Autodesk Fusion 360 part; units mm, degrees
note: some values were not read from the file. Chosen so that the rebuilt part matches the saved one: a direction. Set by a fixed rule: which sketch regions a step uses.
(part 6 of 6)
  spline S38 degree 5 poles (-15.5097, -25.0741) (-15.5106, -25.0685) (-15.5125, -25.0573) (-15.5158, -25.0407) (-15.521, -25.0187) (-15.5286, -24.9914) (-15.537, -24.9643) (-15.5458, -24.9373) (-15.5549, -24.9103) (-15.5642, -24.8833) (-15.5737, -24.8564) (-15.5835, -24.8296) (-15.5935, -24.8028) (-15.604, -24.776) (-15.6148, -24.7494) (-15.6259, -24.7229) (-15.6374, -24.6964) (-15.6491, -24.67) (-15.661, -24.6436) (-15.6731, -24.6173) (-15.6855, -24.591) (-15.698, -24.5648) (-15.7108, -24.5387) (-15.7238, -24.5126) (-15.7371, -24.4866) (-15.7506, -24.4606) (-15.7643, -24.4347) (-15.7782, -24.4088) (-15.7922, -24.383) (-15.8065, -24.3573) (-15.821, -24.3316) (-15.8356, -24.3059) (-15.8505, -24.2803) (-15.8655, -24.2548) (-15.8807, -24.2293) (-15.8961, -24.2039) (-15.9116, -24.1785) (-15.9274, -24.1532) (-15.9433, -24.128) (-15.9594, -24.1028) (-15.9756, -24.0776) (-15.9921, -24.0525) (-16.0086, -24.0275) (-16.0254, -24.0025) (-16.0423, -23.9776) (-16.0594, -23.9527) (-16.0766, -23.9279) (-16.094, -23.9031) (-16.1115, -23.8784) (-16.1292, -23.8537) (-16.1471, -23.8291) (-16.1651, -23.8045) (-16.1832, -23.78) (-16.2015, -23.7556) (-16.22, -23.7312) (-16.2386, -23.7069) (-16.2573, -23.6826) (-16.2762, -23.6584) (-16.2952, -23.6342) (-16.3144, -23.6101) (-16.3337, -23.5861) (-16.3532, -23.5621) (-16.3728, -23.5381) (-16.3925, -23.5143) (-16.4124, -23.4904) (-16.4324, -23.4667) (-16.4525, -23.4429) (-16.4728, -23.4193) (-16.4932, -23.3957) (-16.5137, -23.3722) (-16.5344, -23.3487) (-16.5511, -23.3299) (-16.5636, -23.3159) (-16.572, -23.3066) (-16.5762, -23.3019) knots 0 0 0 0 0 0 0.01428571 0.02857143 0.04285714 0.05714286 0.07142857 0.08571429 0.1 0.11428571 0.12857143 0.14285714 0.15714286 0.17142857 0.18571429 0.2 0.21428571 0.22857143 0.24285714 0.25714286 0.27142857 0.28571429 0.3 0.31428571 0.32857143 0.34285714 0.35714286 0.37142857 0.38571429 0.4 0.41428571 0.42857143 0.44285714 0.45714286 0.47142857 0.48571429 0.5 0.51428571 0.52857143 0.54285714 0.55714286 0.57142857 0.58571429 0.6 0.61428571 0.62857143 0.64285714 0.65714286 0.67142857 0.68571429 0.7 0.71428571 0.72857143 0.74285714 0.75714286 0.77142857 0.78571429 0.8 0.81428571 0.82857143 0.84285714 0.85714286 0.87142857 0.88571429 0.9 0.91428571 0.92857143 0.94285714 0.95714286 0.97142857 0.98571429 1 1 1 1 1 1
  arc A78 (-16.5762, -23.3019) -> (-17.3581, -23.4928) centre (-13.5, -37.5997) ccw
  spline S39 degree 5 poles (-17.3581, -23.4928) (-17.3597, -23.4989) (-17.3628, -23.511) (-17.3675, -23.5292) (-17.3736, -23.5535) (-17.3812, -23.5839) (-17.3885, -23.6143) (-17.3958, -23.6446) (-17.4029, -23.675) (-17.4098, -23.7053) (-17.4166, -23.7356) (-17.4233, -23.7659) (-17.4298, -23.7962) (-17.4361, -23.8265) (-17.4424, -23.8567) (-17.4484, -23.887) (-17.4543, -23.9172) (-17.4601, -23.9474) (-17.4657, -23.9776) (-17.4711, -24.0078) (-17.4764, -24.0379) (-17.4815, -24.0681) (-17.4865, -24.0982) (-17.4914, -24.1283) (-17.496, -24.1584) (-17.5005, -24.1885) (-17.5049, -24.2185) (-17.509, -24.2485) (-17.5131, -24.2785) (-17.5169, -24.3085) (-17.5206, -24.3384) (-17.5241, -24.3684) (-17.5275, -24.3983) (-17.5306, -24.4281) (-17.5337, -24.458) (-17.5365, -24.4878) (-17.5391, -24.5176) (-17.5416, -24.5473) (-17.5439, -24.577) (-17.5461, -24.6067) (-17.548, -24.6364) (-17.5498, -24.666) (-17.5513, -24.6956) (-17.5527, -24.7251) (-17.5539, -24.7546) (-17.5549, -24.7841) (-17.5557, -24.8135) (-17.5563, -24.8429) (-17.5567, -24.8723) (-17.5569, -24.9016) (-17.5569, -24.9308) (-17.5567, -24.96) (-17.5562, -24.9892) (-17.5555, -25.0183) (-17.5546, -25.0473) (-17.5535, -25.0763) (-17.5521, -25.1053) (-17.5505, -25.1342) (-17.5488, -25.163) (-17.5467, -25.1918) (-17.5444, -25.2205) (-17.5417, -25.2491) (-17.5387, -25.2776) (-17.5352, -25.306) (-17.5315, -25.3344) (-17.5275, -25.3626) (-17.5234, -25.3908) (-17.519, -25.419) (-17.5144, -25.447) (-17.5093, -25.475) (-17.5035, -25.5027) (-17.498, -25.5246) (-17.4933, -25.5409) (-17.4899, -25.5517) (-17.4881, -25.557) knots -1 -1 -1 -1 -1 -1 -0.98571429 -0.97142857 -0.95714286 -0.94285714 -0.92857143 -0.91428571 -0.9 -0.88571429 -0.87142857 -0.85714286 -0.84285714 -0.82857143 -0.81428571 -0.8 -0.78571429 -0.77142857 -0.75714286 -0.74285714 -0.72857143 -0.71428571 -0.7 -0.68571429 -0.67142857 -0.65714286 -0.64285714 -0.62857143 -0.61428571 -0.6 -0.58571429 -0.57142857 -0.55714286 -0.54285714 -0.52857143 -0.51428571 -0.5 -0.48571429 -0.47142857 -0.45714286 -0.44285714 -0.42857143 -0.41428571 -0.4 -0.38571429 -0.37142857 -0.35714286 -0.34285714 -0.32857143 -0.31428571 -0.3 -0.28571429 -0.27142857 -0.25714286 -0.24285714 -0.22857143 -0.21428571 -0.2 -0.18571429 -0.17142857 -0.15714286 -0.14285714 -0.12857143 -0.11428571 -0.1 -0.08571429 -0.07142857 -0.05714286 -0.04285714 -0.02857143 -0.01428571 0 0 0 0 0 0
  line L39 (-17.4881, -25.557) -> (-17.3355, -26.0197)
  arc A79 (-17.3983, -26.1457) -> (-17.3355, -26.0197) centre (-17.4305, -26.0511) ccw
  arc A80 (-17.3983, -26.1457) -> (-18.3521, -26.516) centre (-13.5, -37.5997) ccw
  arc A81 (-18.4834, -26.4654) -> (-18.3521, -26.516) centre (-18.3922, -26.4244) ccw
  line L40 (-18.4834, -26.4654) -> (-18.6831, -26.021)
  spline S40 degree 5 poles (-18.6831, -26.021) (-18.6854, -26.0158) (-18.6901, -26.0056) (-18.6976, -25.9904) (-18.7084, -25.9705) (-18.7227, -25.9461) (-18.7378, -25.922) (-18.7534, -25.8982) (-18.7692, -25.8745) (-18.7851, -25.8509) (-18.8013, -25.8274) (-18.8176, -25.8039) (-18.8343, -25.7806) (-18.8513, -25.7575) (-18.8686, -25.7346) (-18.8862, -25.7119) (-18.9042, -25.6893) (-18.9223, -25.6668) (-18.9407, -25.6444) (-18.9592, -25.6221) (-18.9779, -25.5999) (-18.9968, -25.5779) (-19.0159, -25.5559) (-19.0353, -25.5341) (-19.0548, -25.5124) (-19.0745, -25.4908) (-19.0945, -25.4693) (-19.1146, -25.4479) (-19.1349, -25.4266) (-19.1553, -25.4055) (-19.1759, -25.3844) (-19.1967, -25.3634) (-19.2177, -25.3425) (-19.2388, -25.3218) (-19.2601, -25.3011) (-19.2815, -25.2805) (-19.3031, -25.26) (-19.3249, -25.2397) (-19.3468, -25.2194) (-19.3689, -25.1992) (-19.3911, -25.1791) (-19.4134, -25.1591) (-19.4359, -25.1392) (-19.4586, -25.1194) (-19.4814, -25.0997) (-19.5043, -25.0801) (-19.5274, -25.0606) (-19.5506, -25.0412) (-19.5739, -25.0218) (-19.5974, -25.0026) (-19.621, -24.9834) (-19.6447, -24.9644) (-19.6686, -24.9454) (-19.6926, -24.9265) (-19.7167, -24.9078) (-19.741, -24.8891) (-19.7654, -24.8705) (-19.7899, -24.852) (-19.8145, -24.8336) (-19.8393, -24.8152) (-19.8642, -24.797) (-19.8892, -24.7789) (-19.9143, -24.7608) (-19.9395, -24.7428) (-19.9649, -24.725) (-19.9904, -24.7072) (-20.0159, -24.6895) (-20.0417, -24.6719) (-20.0675, -24.6544) (-20.0934, -24.637) (-20.1195, -24.6196) (-20.1404, -24.6058) (-20.1561, -24.5955) (-20.1666, -24.5887) (-20.1719, -24.5853) knots 0 0 0 0 0 0 0.01428571 0.02857143 0.04285714 0.05714286 0.07142857 0.08571429 0.1 0.11428571 0.12857143 0.14285714 0.15714286 0.17142857 0.18571429 0.2 0.21428571 0.22857143 0.24285714 0.25714286 0.27142857 0.28571429 0.3 0.31428571 0.32857143 0.34285714 0.35714286 0.37142857 0.38571429 0.4 0.41428571 0.42857143 0.44285714 0.45714286 0.47142857 0.48571429 0.5 0.51428571 0.52857143 0.54285714 0.55714286 0.57142857 0.58571429 0.6 0.61428571 0.62857143 0.64285714 0.65714286 0.67142857 0.68571429 0.7 0.71428571 0.72857143 0.74285714 0.75714286 0.77142857 0.78571429 0.8 0.81428571 0.82857143 0.84285714 0.85714286 0.87142857 0.88571429 0.9 0.91428571 0.92857143 0.94285714 0.95714286 0.97142857 0.98571429 1 1 1 1 1 1
  arc A82 (-20.1719, -24.5853) -> (-20.8778, -24.972) centre (-13.5, -37.5997) ccw
  spline S41 degree 5 poles (-20.8778, -24.972) (-20.8777, -24.9783) (-20.8776, -24.9909) (-20.8774, -25.0097) (-20.8771, -25.0347) (-20.8765, -25.066) (-20.8757, -25.0972) (-20.8749, -25.1284) (-20.8739, -25.1596) (-20.8727, -25.1907) (-20.8715, -25.2217) (-20.8701, -25.2527) (-20.8685, -25.2836) (-20.8668, -25.3145) (-20.865, -25.3454) (-20.863, -25.3761) (-20.8609, -25.4069) (-20.8586, -25.4375) (-20.8562, -25.4682) (-20.8537, -25.4987) (-20.851, -25.5292) (-20.8481, -25.5597) (-20.8451, -25.5901) (-20.842, -25.6204) (-20.8387, -25.6507) (-20.8353, -25.6809) (-20.8317, -25.711) (-20.828, -25.7411) (-20.8241, -25.7711) (-20.8201, -25.801) (-20.8159, -25.8309) (-20.8115, -25.8607) (-20.807, -25.8905) (-20.8024, -25.9201) (-20.7975, -25.9497) (-20.7926, -25.9793) (-20.7874, -26.0087) (-20.7821, -26.0381) (-20.7767, -26.0674) (-20.771, -26.0966) (-20.7652, -26.1258) (-20.7593, -26.1549) (-20.7531, -26.1838) (-20.7468, -26.2127) (-20.7403, -26.2415) (-20.7337, -26.2703) (-20.7268, -26.2989) (-20.7198, -26.3274) (-20.7126, -26.3559) (-20.7052, -26.3843) (-20.6976, -26.4125) (-20.6899, -26.4407) (-20.6819, -26.4687) (-20.6737, -26.4966) (-20.6652, -26.5245) (-20.6566, -26.5522) (-20.6478, -26.5798) (-20.6388, -26.6073) (-20.6297, -26.6347) (-20.6202, -26.6619) (-20.6106, -26.6891) (-20.6006, -26.716) (-20.5902, -26.7428) (-20.5796, -26.7693) (-20.5686, -26.7957) (-20.5575, -26.822) (-20.5462, -26.8482) (-20.5347, -26.8742) (-20.523, -26.9001) (-20.5108, -26.9258) (-20.498, -26.951) (-20.487, -26.9708) (-20.4782, -26.9853) (-20.4722, -26.9948) (-20.4691, -26.9996) knots -1 -1 -1 -1 -1 -1 -0.98571429 -0.97142857 -0.95714286 -0.94285714 -0.92857143 -0.91428571 -0.9 -0.88571429 -0.87142857 -0.85714286 -0.84285714 -0.82857143 -0.81428571 -0.8 -0.78571429 -0.77142857 -0.75714286 -0.74285714 -0.72857143 -0.71428571 -0.7 -0.68571429 -0.67142857 -0.65714286 -0.64285714 -0.62857143 -0.61428571 -0.6 -0.58571429 -0.57142857 -0.55714286 -0.54285714 -0.52857143 -0.51428571 -0.5 -0.48571429 -0.47142857 -0.45714286 -0.44285714 -0.42857143 -0.41428571 -0.4 -0.38571429 -0.37142857 -0.35714286 -0.34285714 -0.32857143 -0.31428571 -0.3 -0.28571429 -0.27142857 -0.25714286 -0.24285714 -0.22857143 -0.21428571 -0.2 -0.18571429 -0.17142857 -0.15714286 -0.14285714 -0.12857143 -0.11428571 -0.1 -0.08571429 -0.07142857 -0.05714286 -0.04285714 -0.02857143 -0.01428571 0 0 0 0 0 0
  line L41 (-20.4691, -26.9996) -> (-20.202, -27.407)
  arc A83 (-20.23, -27.545) -> (-20.202, -27.407) centre (-20.2856, -27.4619) ccw
  arc A84 (-20.23, -27.545) -> (-21.0554, -28.1495) centre (-13.5, -37.5997) ccw
  arc A85 (-21.1954, -28.1346) -> (-21.0554, -28.1495) centre (-21.1179, -28.0714) ccw
  line L42 (-21.1954, -28.1346) -> (-21.5032, -27.757)
  spline S42 degree 5 poles (-21.5032, -27.757) (-21.5068, -27.7526) (-21.5141, -27.7439) (-21.5253, -27.7312) (-21.5408, -27.7148) (-21.561, -27.6949) (-21.5818, -27.6756) (-21.6029, -27.6566) (-21.6243, -27.6378) (-21.6459, -27.6191) (-21.6675, -27.6006) (-21.6894, -27.5822) (-21.7115, -27.564) (-21.7339, -27.5461) (-21.7566, -27.5284) (-21.7795, -27.511) (-21.8027, -27.4938) (-21.826, -27.4768) (-21.8495, -27.4599) (-21.8732, -27.4432) (-21.897, -27.4266) (-21.921, -27.4102) (-21.9452, -27.3939) (-21.9695, -27.3779) (-21.994, -27.3619) (-22.0186, -27.3462) (-22.0434, -27.3306) (-22.0684, -27.3151) (-22.0935, -27.2998) (-22.1187, -27.2847) (-22.1441, -27.2697) (-22.1696, -27.2548) (-22.1952, -27.24) (-22.221, -27.2254) (-22.2469, -27.211) (-22.273, -27.1967) (-22.2991, -27.1825) (-22.3254, -27.1684) (-22.3518, -27.1545) (-22.3784, -27.1407) (-22.405, -27.1271) (-22.4318, -27.1135) (-22.4587, -27.1001) (-22.4857, -27.0869) (-22.5128, -27.0737) (-22.54, -27.0607) (-22.5673, -27.0478) (-22.5948, -27.0351) (-22.6223, -27.0224) (-22.65, -27.0099) (-22.6778, -26.9976) (-22.7056, -26.9853) (-22.7336, -26.9732) (-22.7617, -26.9611) (-22.7898, -26.9492) (-22.8181, -26.9375) (-22.8465, -26.9258) (-22.8749, -26.9143) (-22.9035, -26.9029) (-22.9321, -26.8916) (-22.9609, -26.8804) (-22.9897, -26.8694) (-23.0187, -26.8584) (-23.0477, -26.8476) (-23.0768, -26.8369) (-23.106, -26.8263) (-23.1353, -26.8158) (-23.1647, -26.8055) (-23.1942, -26.7953) (-23.2237, -26.7852) (-23.2534, -26.7752) (-23.2772, -26.7672) (-23.2951, -26.7614) (-23.307, -26.7575) (-23.313, -26.7555) knots 0 0 0 0 0 0 0.01428571 0.02857143 0.04285714 0.05714286 0.07142857 0.08571429 0.1 0.11428571 0.12857143 0.14285714 0.15714286 0.17142857 0.18571429 0.2 0.21428571 0.22857143 0.24285714 0.25714286 0.27142857 0.28571429 0.3 0.31428571 0.32857143 0.34285714 0.35714286 0.37142857 0.38571429 0.4 0.41428571 0.42857143 0.44285714 0.45714286 0.47142857 0.48571429 0.5 0.51428571 0.52857143 0.54285714 0.55714286 0.57142857 0.58571429 0.6 0.61428571 0.62857143 0.64285714 0.65714286 0.67142857 0.68571429 0.7 0.71428571 0.72857143 0.74285714 0.75714286 0.77142857 0.78571429 0.8 0.81428571 0.82857143 0.84285714 0.85714286 0.87142857 0.88571429 0.9 0.91428571 0.92857143 0.94285714 0.95714286 0.97142857 0.98571429 1 1 1 1 1 1
  arc A86 (-23.313, -26.7555) -> (-23.8947, -27.3118) centre (-13.5, -37.5997) ccw
  spline S43 degree 5 poles (-23.8947, -27.3118) (-23.893, -27.3179) (-23.8897, -27.33) (-23.8846, -27.3481) (-23.8777, -27.3722) (-23.8691, -27.4023) (-23.8603, -27.4322) (-23.8514, -27.4621) (-23.8424, -27.492) (-23.8332, -27.5217) (-23.824, -27.5514) (-23.8146, -27.5809) (-23.8051, -27.6104) (-23.7954, -27.6398) (-23.7857, -27.6691) (-23.7758, -27.6983) (-23.7658, -27.7275) (-23.7557, -27.7565) (-23.7454, -27.7855) (-23.7351, -27.8143) (-23.7246, -27.8431) (-23.7139, -27.8718) (-23.7032, -27.9003) (-23.6923, -27.9288) (-23.6813, -27.9572) (-23.6702, -27.9855) (-23.6589, -28.0137) (-23.6475, -28.0418) (-23.636, -28.0698) (-23.6244, -28.0976) (-23.6126, -28.1254) (-23.6007, -28.1531) (-23.5886, -28.1807) (-23.5764, -28.2081) (-23.5641, -28.2355) (-23.5517, -28.2627) (-23.5391, -28.2898) (-23.5264, -28.3168) (-23.5135, -28.3437) (-23.5005, -28.3705) (-23.4874, -28.3971) (-23.4741, -28.4237) (-23.4606, -28.4501) (-23.4471, -28.4763) (-23.4333, -28.5025) (-23.4195, -28.5285) (-23.4054, -28.5544) (-23.3913, -28.5802) (-23.377, -28.6058) (-23.3625, -28.6313) (-23.3478, -28.6566) (-23.333, -28.6818) (-23.3181, -28.7068) (-23.3029, -28.7316) (-23.2876, -28.7563) (-23.2721, -28.7809) (-23.2564, -28.8053) (-23.2406, -28.8295) (-23.2247, -28.8536) (-23.2085, -28.8775) (-23.1922, -28.9012) (-23.1755, -28.9246) (-23.1586, -28.9478) (-23.1415, -28.9707) (-23.1241, -28.9934) (-23.1065, -29.0158) (-23.0888, -29.0382) (-23.0709, -29.0604) (-23.0529, -29.0824) (-23.0346, -29.104) (-23.0156, -29.1251) (-22.9999, -29.1413) (-22.9877, -29.1531) (-22.9793, -29.1607) (-22.9751, -29.1645) knots -1 -1 -1 -1 -1 -1 -0.98571429 -0.97142857 -0.95714286 -0.94285714 -0.92857143 -0.91428571 -0.9 -0.88571429 -0.87142857 -0.85714286 -0.84285714 -0.82857143 -0.81428571 -0.8 -0.78571429 -0.77142857 -0.75714286 -0.74285714 -0.72857143 -0.71428571 -0.7 -0.68571429 -0.67142857 -0.65714286 -0.64285714 -0.62857143 -0.61428571 -0.6 -0.58571429 -0.57142857 -0.55714286 -0.54285714 -0.52857143 -0.51428571 -0.5 -0.48571429 -0.47142857 -0.45714286 -0.44285714 -0.42857143 -0.41428571 -0.4 -0.38571429 -0.37142857 -0.35714286 -0.34285714 -0.32857143 -0.31428571 -0.3 -0.28571429 -0.27142857 -0.25714286 -0.24285714 -0.22857143 -0.21428571 -0.2 -0.18571429 -0.17142857 -0.15714286 -0.14285714 -0.12857143 -0.11428571 -0.1 -0.08571429 -0.07142857 -0.05714286 -0.04285714 -0.02857143 -0.01428571 0 0 0 0 0 0
  line L43 (-22.9751, -29.1645) -> (-22.6117, -29.4889)
  arc A87 (-22.603, -29.6294) -> (-22.6117, -29.4889) centre (-22.6783, -29.5635) ccw
  arc A88 (-22.603, -29.6294) -> (-23.2439, -30.427) centre (-13.5, -37.5997) ccw
  arc A89 (-23.3829, -30.4488) -> (-23.2439, -30.427) centre (-23.3244, -30.3677) ccw
  line L44 (-23.3829, -30.4488) -> (-23.778, -30.1638)
  spline S44 degree 5 poles (-23.778, -30.1638) (-23.7826, -30.1605) (-23.7919, -30.154) (-23.806, -30.1446) (-23.8252, -30.1327) (-23.8498, -30.1187) (-23.8749, -30.1055) (-23.9003, -30.0926) (-23.9258, -30.08) (-23.9515, -30.0675) (-23.9772, -30.0552) (-24.0031, -30.0431) (-24.0292, -30.0312) (-24.0554, -30.0197) (-24.0819, -30.0085) (-24.1085, -29.9977) (-24.1354, -29.987) (-24.1623, -29.9766) (-24.1894, -29.9664) (-24.2166, -29.9564) (-24.2439, -29.9466) (-24.2713, -29.9369) (-24.2988, -29.9275) (-24.3265, -29.9182) (-24.3543, -29.9092) (-24.3822, -29.9003) (-24.4102, -29.8917) (-24.4383, -29.8832) (-24.4665, -29.875) (-24.4948, -29.8668) (-24.5232, -29.8589) (-24.5517, -29.8511) (-24.5802, -29.8435) (-24.6089, -29.8361) (-24.6377, -29.8288) (-24.6665, -29.8217) (-24.6955, -29.8148) (-24.7245, -29.808) (-24.7536, -29.8014) (-24.7828, -29.795) (-24.8121, -29.7887) (-24.8415, -29.7826) (-24.8709, -29.7766) (-24.9004, -29.7707) (-24.93, -29.7651) (-24.9597, -29.7596) (-24.9894, -29.7542) (-25.0192, -29.749) (-25.0491, -29.7439) (-25.079, -29.739) (-25.1091, -29.7342) (-25.1392, -29.7296) (-25.1693, -29.7251) (-25.1995, -29.7207) (-25.2298, -29.7165) (-25.2602, -29.7125) (-25.2906, -29.7086) (-25.3211, -29.7048) (-25.3516, -29.7012) (-25.3822, -29.6977) (-25.4129, -29.6943) (-25.4436, -29.6911) (-25.4744, -29.688) (-25.5052, -29.6851) (-25.5361, -29.6823) (-25.5671, -29.6796) (-25.5981, -29.6771) (-25.6291, -29.6747) (-25.6603, -29.6725) (-25.6914, -29.6703) (-25.7227, -29.6684) (-25.7477, -29.6669) (-25.7665, -29.6658) (-25.779, -29.6651) (-25.7853, -29.6648) knots 0 0 0 0 0 0 0.01428571 0.02857143 0.04285714 0.05714286 0.07142857 0.08571429 0.1 0.11428571 0.12857143 0.14285714 0.15714286 0.17142857 0.18571429 0.2 0.21428571 0.22857143 0.24285714 0.25714286 0.27142857 0.28571429 0.3 0.31428571 0.32857143 0.34285714 0.35714286 0.37142857 0.38571429 0.4 0.41428571 0.42857143 0.44285714 0.45714286 0.47142857 0.48571429 0.5 0.51428571 0.52857143 0.54285714 0.55714286 0.57142857 0.58571429 0.6 0.61428571 0.62857143 0.64285714 0.65714286 0.67142857 0.68571429 0.7 0.71428571 0.72857143 0.74285714 0.75714286 0.77142857 0.78571429 0.8 0.81428571 0.82857143 0.84285714 0.85714286 0.87142857 0.88571429 0.9 0.91428571 0.92857143 0.94285714 0.95714286 0.97142857 0.98571429 1 1 1 1 1 1
  arc A90 (-25.7853, -29.6648) -> (-26.2032, -30.3527) centre (-13.5, -37.5997) ccw
  spline S45 degree 5 poles (-26.2032, -30.3527) (-26.2, -30.3581) (-26.1936, -30.3689) (-26.1841, -30.3851) (-26.1712, -30.4066) (-26.1551, -30.4334) (-26.1388, -30.4601) (-26.1225, -30.4867) (-26.106, -30.5132) (-26.0895, -30.5395) (-26.0729, -30.5658) (-26.0562, -30.5919) (-26.0394, -30.6179) (-26.0224, -30.6438) (-26.0054, -30.6696) (-25.9883, -30.6953) (-25.9711, -30.7208) (-25.9538, -30.7463) (-25.9364, -30.7716) (-25.919, -30.7968) (-25.9014, -30.8218) (-25.8837, -30.8468) (-25.8659, -30.8716) (-25.848, -30.8963) (-25.8301, -30.9209) (-25.812, -30.9453) (-25.7938, -30.9696) (-25.7755, -30.9938) (-25.7572, -31.0179) (-25.7387, -31.0418) (-25.7201, -31.0656) (-25.7015, -31.0892) (-25.6827, -31.1127) (-25.6638, -31.1361) (-25.6448, -31.1593) (-25.6258, -31.1824) (-25.6066, -31.2053) (-25.5873, -31.2281) (-25.5679, -31.2508) (-25.5484, -31.2733) (-25.5288, -31.2956) (-25.5091, -31.3178) (-25.4893, -31.3398) (-25.4694, -31.3617) (-25.4494, -31.3834) (-25.4293, -31.405) (-25.409, -31.4263) (-25.3887, -31.4475) (-25.3682, -31.4686) (-25.3476, -31.4895) (-25.3269, -31.5101) (-25.3061, -31.5306) (-25.2852, -31.5509) (-25.2641, -31.571) (-25.2429, -31.5909) (-25.2216, -31.6106) (-25.2002, -31.6301) (-25.1786, -31.6494) (-25.157, -31.6685) (-25.1352, -31.6875) (-25.1133, -31.7061) (-25.0911, -31.7244) (-25.0688, -31.7424) (-25.0463, -31.7601) (-25.0236, -31.7775) (-25.0008, -31.7947) (-24.9779, -31.8117) (-24.955, -31.8285) (-24.9319, -31.8451) (-24.9085, -31.8613) (-24.8848, -31.8767) (-24.8654, -31.8883) (-24.8505, -31.8965) (-24.8405, -31.9017) (-24.8355, -31.9043) knots -1 -1 -1 -1 -1 -1 -0.98571429 -0.97142857 -0.95714286 -0.94285714 -0.92857143 -0.91428571 -0.9 -0.88571429 -0.87142857 -0.85714286 -0.84285714 -0.82857143 -0.81428571 -0.8 -0.78571429 -0.77142857 -0.75714286 -0.74285714 -0.72857143 -0.71428571 -0.7 -0.68571429 -0.67142857 -0.65714286 -0.64285714 -0.62857143 -0.61428571 -0.6 -0.58571429 -0.57142857 -0.55714286 -0.54285714 -0.52857143 -0.51428571 -0.5 -0.48571429 -0.47142857 -0.45714286 -0.44285714 -0.42857143 -0.41428571 -0.4 -0.38571429 -0.37142857 -0.35714286 -0.34285714 -0.32857143 -0.31428571 -0.3 -0.28571429 -0.27142857 -0.25714286 -0.24285714 -0.22857143 -0.21428571 -0.2 -0.18571429 -0.17142857 -0.15714286 -0.14285714 -0.12857143 -0.11428571 -0.1 -0.08571429 -0.07142857 -0.05714286 -0.04285714 -0.02857143 -0.01428571 0 0 0 0 0 0
  line L45 (-24.8355, -31.9043) -> (-24.4004, -32.1236)
  arc A91 (-24.3557, -32.257) -> (-24.4004, -32.1236) centre (-24.4454, -32.2129) ccw
  arc A92 (-24.3557, -32.257) -> (-24.7683, -33.1933) centre (-13.5, -37.5997) ccw
  arc A93 (-24.8969, -33.2504) -> (-24.7683, -33.1933) centre (-24.8614, -33.1569) ccw
  line L46 (-24.8969, -33.2504) -> (-25.3524, -33.0773)
  spline S46 degree 5 poles (-25.3524, -33.0773) (-25.3577, -33.0753) (-25.3683, -33.0714) (-25.3843, -33.066) (-25.406, -33.0595) (-25.4334, -33.0524) (-25.4611, -33.0461) (-25.4889, -33.0402) (-25.5168, -33.0346) (-25.5448, -33.0292) (-25.5729, -33.024) (-25.601, -33.019) (-25.6293, -33.0143) (-25.6576, -33.01) (-25.6861, -33.006) (-25.7146, -33.0024) (-25.7433, -32.9991) (-25.772, -32.996) (-25.8008, -32.9931) (-25.8297, -32.9905) (-25.8586, -32.9881) (-25.8876, -32.9858) (-25.9166, -32.9838) (-25.9457, -32.9821) (-25.9749, -32.9805) (-26.0041, -32.9792) (-26.0334, -32.9781) (-26.0627, -32.9772) (-26.0921, -32.9765) (-26.1215, -32.976) (-26.151, -32.9757) (-26.1806, -32.9755) (-26.2101, -32.9756) (-26.2398, -32.9758) (-26.2694, -32.9763) (-26.2991, -32.9769) (-26.3289, -32.9777) (-26.3587, -32.9787) (-26.3885, -32.9798) (-26.4184, -32.9811) (-26.4483, -32.9826) (-26.4782, -32.9843) (-26.5082, -32.9861) (-26.5382, -32.9882) (-26.5683, -32.9903) (-26.5984, -32.9927) (-26.6285, -32.9952) (-26.6586, -32.9979) (-26.6888, -33.0007) (-26.719, -33.0037) (-26.7492, -33.0068) (-26.7795, -33.0102) (-26.8098, -33.0136) (-26.8401, -33.0173) (-26.8705, -33.021) (-26.9008, -33.025) (-26.9312, -33.0291) (-26.9616, -33.0333) (-26.9921, -33.0377) (-27.0225, -33.0423) (-27.053, -33.047) (-27.0835, -33.0518) (-27.1141, -33.0568) (-27.1446, -33.062) (-27.1752, -33.0673) (-27.2058, -33.0727) (-27.2364, -33.0783) (-27.267, -33.084) (-27.2976, -33.0899) (-27.3283, -33.0959) (-27.359, -33.1021) (-27.3835, -33.1071) (-27.4019, -33.111) (-27.4142, -33.1136) (-27.4204, -33.1149) knots 0 0 0 0 0 0 0.01428571 0.02857143 0.04285714 0.05714286 0.07142857 0.08571429 0.1 0.11428571 0.12857143 0.14285714 0.15714286 0.17142857 0.18571429 0.2 0.21428571 0.22857143 0.24285714 0.25714286 0.27142857 0.28571429 0.3 0.31428571 0.32857143 0.34285714 0.35714286 0.37142857 0.38571429 0.4 0.41428571 0.42857143 0.44285714 0.45714286 0.47142857 0.48571429 0.5 0.51428571 0.52857143 0.54285714 0.55714286 0.57142857 0.58571429 0.6 0.61428571 0.62857143 0.64285714 0.65714286 0.67142857 0.68571429 0.7 0.71428571 0.72857143 0.74285714 0.75714286 0.77142857 0.78571429 0.8 0.81428571 0.82857143 0.84285714 0.85714286 0.87142857 0.88571429 0.9 0.91428571 0.92857143 0.94285714 0.95714286 0.97142857 0.98571429 1 1 1 1 1 1
  arc A94 (-27.4204, -33.1149) -> (-27.646, -33.8875) centre (-13.5, -37.5997) ccw
  spline S47 degree 5 poles (-27.646, -33.8875) (-27.6415, -33.8919) (-27.6326, -33.9007) (-27.6191, -33.9138) (-27.6012, -33.9313) (-27.5786, -33.953) (-27.556, -33.9746) (-27.5334, -33.996) (-27.5106, -34.0173) (-27.4878, -34.0385) (-27.465, -34.0596) (-27.4421, -34.0805) (-27.4191, -34.1012) (-27.3961, -34.1219) (-27.373, -34.1424) (-27.3498, -34.1628) (-27.3266, -34.183) (-27.3033, -34.2031) (-27.2799, -34.223) (-27.2565, -34.2428) (-27.233, -34.2625) (-27.2095, -34.282) (-27.1859, -34.3014) (-27.1622, -34.3206) (-27.1385, -34.3397) (-27.1147, -34.3586) (-27.0909, -34.3774) (-27.067, -34.3961) (-27.043, -34.4145) (-27.019, -34.4329) (-26.9949, -34.451) (-26.9707, -34.469) (-26.9465, -34.4869) (-26.9223, -34.5046) (-26.8979, -34.5221) (-26.8735, -34.5394) (-26.8491, -34.5566) (-26.8245, -34.5737) (-26.7999, -34.5905) (-26.7753, -34.6072) (-26.7506, -34.6237) (-26.7258, -34.6401) (-26.701, -34.6562) (-26.6761, -34.6722) (-26.6511, -34.688) (-26.6261, -34.7036) (-26.601, -34.719) (-26.5759, -34.7342) (-26.5507, -34.7492) (-26.5254, -34.7641) (-26.5, -34.7787) (-26.4746, -34.7931) (-26.4492, -34.8072) (-26.4236, -34.8212) (-26.398, -34.8349) (-26.3723, -34.8484) (-26.3466, -34.8617) (-26.3207, -34.8748) (-26.2949, -34.8877) (-26.2689, -34.9003) (-26.2429, -34.9126) (-26.2168, -34.9246) (-26.1906, -34.9362) (-26.1643, -34.9475) (-26.1379, -34.9584) (-26.1114, -34.9691) (-26.0849, -34.9796) (-26.0583, -34.9899) (-26.0317, -35) (-26.005, -35.0095) (-25.9781, -35.0183) (-25.9563, -35.0245) (-25.9399, -35.0286) (-25.9288, -35.031) (-25.9233, -35.0322) knots -1 -1 -1 -1 -1 -1 -0.98571429 -0.97142857 -0.95714286 -0.94285714 -0.92857143 -0.91428571 -0.9 -0.88571429 -0.87142857 -0.85714286 -0.84285714 -0.82857143 -0.81428571 -0.8 -0.78571429 -0.77142857 -0.75714286 -0.74285714 -0.72857143 -0.71428571 -0.7 -0.68571429 -0.67142857 -0.65714286 -0.64285714 -0.62857143 -0.61428571 -0.6 -0.58571429 -0.57142857 -0.55714286 -0.54285714 -0.52857143 -0.51428571 -0.5 -0.48571429 -0.47142857 -0.45714286 -0.44285714 -0.42857143 -0.41428571 -0.4 -0.38571429 -0.37142857 -0.35714286 -0.34285714 -0.32857143 -0.31428571 -0.3 -0.28571429 -0.27142857 -0.25714286 -0.24285714 -0.22857143 -0.21428571 -0.2 -0.18571429 -0.17142857 -0.15714286 -0.14285714 -0.12857143 -0.11428571 -0.1 -0.08571429 -0.07142857 -0.05714286 -0.04285714 -0.02857143 -0.01428571 0 0 0 0 0 0
  line L47 (-25.9233, -35.0322) -> (-25.4463, -35.1314)
  arc A95 (-25.3686, -35.2487) -> (-25.4463, -35.1314) centre (-25.4667, -35.2293) ccw
  circle A96 centre (-13.5, -37.5997) radius 1.5
  line L48 (-17.5, -37.6105) -> (-17.4165, -68.6105)
  arc A97 (-17.4165, -68.6105) -> (-9.4165, -68.5889) centre (-13.4165, -68.5997) ccw
  line L49 (-9.4165, -68.5889) -> (-9.5, -37.5889)
  arc A98 (-9.5, -37.5889) -> (-17.5, -37.6105) centre (-13.5, -37.5997) ccw
  line L50 (-13.5, -37.5997) -> (-13.4165, -68.5997) construction
  circle A99 centre (-13.4165, -68.5997) radius 1.5
  dimension "d71" = 31
  dimension "d72" = 4
  dimension "d73" = 3
  constraint tangent L48 A97
  constraint tangent A97 L49
  constraint parallel L48 L49
  constraint tangent L49 A98
  constraint tangent L48 A98
  constraint coincident A0.centre A2.centre
  constraint concentric A97 A99
  measures "d71" vertical distance of A0.centre A97.centre
  measures "d72" radius of A97
  measures "d73" diameter of A99
extrude "Extrude3'" add sketch "Sketch6" against normal blind 3 contours A22 S11 L11 A23 A24 A25 L12 S12 A26 S13 L13 A27 A28 A29 L14 S14 A30 S15 L15 A31 A32 L48 L49 A98 | A22 S11 L11 A23 A24 A25 L12 S12 A26 S13 L13 A27 A28 A29 L14 S14 A30 S15 L48 A97 L49 sketch seen with x (0.999391, 0.034899, 0) y (-0.034899, 0.999391, 0) z (0, 0, 1) at (-12.1796, -38.048, -3) bodies 5 in component "Spur Gear (24 teeth) (1)"
mirror "MirrorComponent1" about plane through (0, 0, 0) normal (0, 0, 1) of bodies 1 makes body 6 in component "Component1(Mirror)"
mirror "MirrorComponent1'" about plane through (0, 0, 0) normal (0, 0, 1) of bodies 2 makes body 7 in component "Component2(Mirror)"
sketch "Sketch7" plane through (0, 0, 0) normal (0, 1, 0) x (1, 0, 0)
  line L0 (35, -40) -> (35, -26)
  line L1 (35, -40) -> (32.5, -40)
  line L2 (32.5, -40) -> (32.5, -39)
  line L3 (32.5, -39) -> (33.5, -39)
  line L4 (33.5, -39) -> (33.5, -27)
  line L5 (33.5, -27) -> (32.5, -27)
  line L6 (32.5, -27) -> (32.5, -26)
  line L7 (32.5, -26) -> (35, -26)
  dimension "d127" = 14
  dimension "d128" = 1
  dimension "d129" = 1
  dimension "d130" = 2.5
  dimension "d131" = 1.5
  dimension "d132" = 2.5
  constraint vertical L0
  constraint perpendicular L0 L1
  constraint perpendicular L1 L2
  constraint perpendicular L2 L3
  constraint perpendicular L3 L4
  constraint perpendicular L2 L5
  constraint perpendicular L5 L6
  measures "d127" distance of L0.start L0.end
  measures "d128" distance of L1.end L2.end
  measures "d129" distance of L5.end L6.end
  measures "d130" distance of L0.start L1.end
  measures "d131" distance of L0 L4
  measures "d132" distance of L0.end L6.end
revolve "Revolve1" add sketch "Sketch7" angle 360 about axis through (35, 0, 40) along (0, 0, -1) separate body makes body 8 in component "Component'''"
component "Component" placed x (0.374661, 0.927162, 0) y (-0.927162, 0.374661, 0) z (0, 0, 1) at (-18.2225, 68.2379, 0)
component "Component'" placed x (-0.152909, 0.98824, 0) y (-0.98824, -0.152909, 0) z (0, 0, 1) at (80.3464, -4.6499, 3)
component "Component''" placed x (1, 0, 0) y (0, 1, 0) z (0, 0, 1) at (0, 0, 0)
component "Spur Gear (24 teeth)" placed x (0.675636, 0.737235, 0) y (0.737235, -0.675636, 0) z (0, 0, -1) at (-13.5, 37.5997, 6)
component "Spur Gear (24 teeth) (1)" placed x (0.982987, -0.183674, 0) y (0.183674, 0.982987, 0) z (0, 0, 1) at (13.5, 37.5997, 3)
component "Component1(Mirror)" placed x (-0.37468, 0.927154, 0) y (0.927154, 0.37468, 0) z (0, 0, -1) at (18.4288, 68.2055, 0)
component "Component2(Mirror)" placed x (0.159548, 0.98719, 0) y (0.98719, -0.159548, 0) z (0, 0, -1) at (-80.7656, -4.0731, 3)
component "Component''" placed x (1, 0, 0) y (0, 1, 0) z (0, 0, 1) at (0, 0, -3)
component "Component'" placed x (-0.152909, 0.98824, 0) y (-0.98824, -0.152909, 0) z (0, 0, 1) at (80.3464, -4.6499, -6)
component "Component'" placed x (0.159548, 0.98719, 0) y (-0.98719, 0.159548, 0) z (0, 0, 1) at (67.313, -28.0054, -6)
component "Component" placed x (0.374661, 0.927162, 0) y (-0.927162, 0.374661, 0) z (0, 0, 1) at (-18.2225, 68.2379, -3)
component "Component1(Mirror)" placed x (-0.37468, 0.927154, 0) y (0.927154, 0.37468, 0) z (0, 0, -1) at (18.4288, 68.2055, -3)
component "Component'''" placed x (0.982987, -0.183674, 0) y (0.183674, 0.982987, 0) z (0, 0, 1) at (-20.9046, 44.0283, -33)
component "Component'''" placed x (0.982987, -0.183674, 0) y (0.183674, 0.982987, 0) z (0, 0, 1) at (-20.9046, 44.0283, -33)
